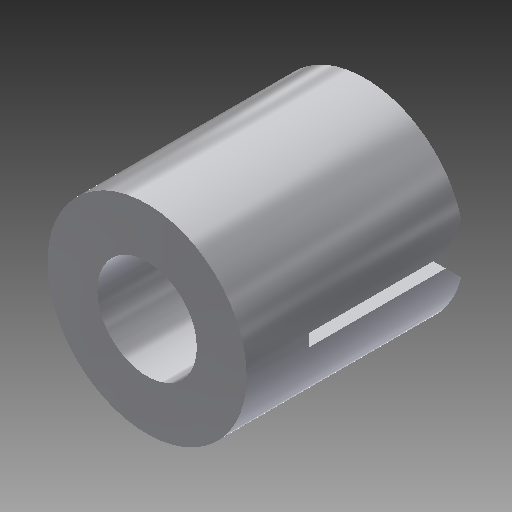
# Autodesk Inventor part: 402-02
Saved by Autodesk Inventor 2019 (Build 230136000, 136)
## iProperties
Company: Autodesk Inc.
Created: 2017-06-27
Part Number: 402-02
Material: PVC-U
Document SubType Name: Modeling
Designer: Autodesk Inc.
Mass: 0.0260113 g
Surface Area: 0.699477 cm^2
Volume: 0.0201638 cm^3
Density: 1.29 g/cm^3
Appearance: Smooth - White
Author: Inventor
Autodesk Inventor part; units mm, degrees
ref_plane "YZ Plane" through (0, 0, 0) normal (1, 0, 0) x (0, 1, 0)
ref_plane "XZ Plane" through (0, 0, 0) normal (0, 1, 0) x (-1, 0, 0)
ref_plane "XY Plane" through (0, 0, 0) normal (0, 0, 1) x (1, 0, 0)
sketch "Sketch1" plane through (0, 0, 0) normal (0, 0, 1) x (1, 0, 0)
  circle A0 centre (0, 0) radius 1.6
  dimension "d0" = 3.2
  constraints: 1 centre point, 1 coincident
  measures "d0" diameter of A0
extrude "Extrusion1" add sketch "Sketch1" along normal blind 3.5
hole "Hole1" at (0, 0, 3.5) direction (0, 0, -1) diameter 1.3 end through all counterbore diameter 1.6 counterbore depth 4
sketch "Sketch2" plane through (0, 0, 0) normal (1, 0, 0) x (0, 1, 0)
  line L0 (-0.1, 0) -> (0.1, 0)
  line L1 (0.1, 0) -> (0.1, 2.5)
  line L2 (0.1, 2.5) -> (-0.1, 2.5)
  line L3 (-0.1, 2.5) -> (-0.1, 0)
  point P0 (0, 0)
  point P1 (0, 0)
  dimension "d14" = 0.2
  dimension "d15" = 2.5
  constraints: 8 end point, 2 parallel, 1 coincident, 1 horizontal, 1 midpoint, 1 perpendicular
  measures "d14" distance of L2.end L1.end
  measures "d15" distance of L1.end L0.end
extrude "Extrusion2" cut sketch "Sketch2" along normal through all both and the other way through all
chamfer "Chamfer1" distance 0.3 angle 45 4 edges at (1.1953, 0.1, 0) (-1.1953, 0.1, 0) (-1.1953, -0.1, 0) (1.1953, -0.1, 0)
body "Solid1"
